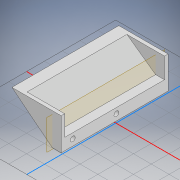
# Autodesk Inventor part: 000.001.007 - Накладка
Saved by Autodesk Inventor 2022 (Build 260153000, 153)
## iProperties
Created: 2022-11-12
Part Number: 000.001.007 - Накладка
Material: Типовые
Document SubType Name: Modeling
Designer: Petrov Ivan
Density: 1 g/cm^3
Appearance: По умолчанию
Author: Petrov Ivan
Autodesk Inventor part; units mm, degrees
ref_plane "YZ Plane" through (0, 0, 0) normal (1, 0, 0) x (0, 1, 0)
ref_plane "XZ Plane" through (0, 0, 0) normal (0, 1, 0) x (-1, 0, 0)
ref_plane "XY Plane" through (0, 0, 0) normal (0, 0, 1) x (1, 0, 0)
sketch "Эскиз1" plane through (0, 0, 0) normal (1, 0, 0) x (0, 1, 0)
  circle A0 centre (-6.0133, 48.1994) radius 2.75 projected
  circle A1 centre (-6.0133, -0.8006) radius 2.75 projected
  line L0 (-13.0133, 61.1994) -> (-13.0133, -18.8006) projected
  line L1 (38.9867, 61.1994) -> (-13.0133, 61.1994) projected
  line L2 (33.9867, -18.8006) -> (-13.0133, -18.8006) projected
  line L3 (-0.0133, 61.1994) -> (-0.0133, -18.8006)
  point P0 (0, 0)
  dimension "d0" = 13
  constraints: 2 end point, 2 point on line, 1 perpendicular
  measures "d0" distance between parallel lines of L0 L3
extrude "Выдавливание1" add sketch "Эскиз1" against normal blind 10
sketch "Эскиз2" plane through (0, -13.0133, 61.1994) normal (0, 0, 1) x (1, 0, 0)
  line L0 (-55.25, 38) -> (-55.25, 36) projected
  line L1 (-10, 13) -> (-10, 0) projected
  line L2 (-10, 0) -> (-55.25, 36)
  line L3 (0, 13) -> (-10, 13) projected
  line L4 (-10, 13) -> (-42.25, 36)
  line L5 (-55.25, 36) -> (-42.25, 36)
  point P0 (0, 13.0133)
  dimension "d3" = 13
  dimension "d4" = 13
  constraints: 6 end point, 1 horizontal
  measures "d3" distance of L1.start L1.end
  measures "d4" distance of L0.end L4.end
extrude "Выдавливание2" add sketch "Эскиз2" against normal up to surface (80 mm away)
sketch "Эскиз3" plane through (0, -13.0133, 61.1994) normal (0, 0, 1) x (1, 0, 0)
  line L0 (0, 13) -> (0, 0) projected
  line L1 (0, 13) -> (0, 36)
  line L2 (-10, 13) -> (-42.25, 36) projected
  line L3 (0, 36) -> (-42.25, 36)
  line L4 (0, 13) -> (-10, 13) projected
  point P0 (0, 13.0133)
  constraints: 4 end point, 1 perpendicular, 1 vertical
extrude "Выдавливание3" add sketch "Эскиз3" against normal blind 4
sketch "Эскиз4" plane through (-10, -6.0133, 48.1994) normal (1, 0, 0) x (0, 0, -1)
  circle A0 centre (49, 0) radius 2.75 projected
  circle A1 centre (0, 0) radius 2.75 projected
  point P0 (48.1994, 6.0133)
extrude "Выдавливание4" cut sketch "Эскиз4" against normal through all
ref_plane "РабПлоскость1" through (-10, -13.0133, 61.1994) normal (1, 0, 0) x (0, 0, 1)
sketch "Эскиз5" plane through (-10, -13.0133, 61.1994) normal (1, 0, 0) x (0, 0, 1)
  circle A0 centre (-13, -7) radius 2.75 projected
  circle A1 centre (-62, -7) radius 2.75 projected
  circle A2 centre (-13, -7) radius 2.75 projected
  circle A3 centre (-13, -7) radius 5
  circle A4 centre (-62, -7) radius 5
  point P0 (-61.1994, -13.0133)
  dimension "d12" = 10
  dimension "d13" = 10
  constraints: 2 centre point, 2 coincident
  measures "d12" diameter of A3
  measures "d13" diameter of A4
extrude "Выдавливание5" cut sketch "Эскиз5" against normal through all contours A0 | A1 | A3 | A4
move faces "Перенос2" translate (0, 0, -40) faces at (-35.8333, 10.9867, -18.8006)
sketch "Эскиз6" plane through (0, -13.0133, -58.8006) normal (0, 0, -1) x (-1, 0, 0)
  line L0 (42.25, 36) -> (10, 13) projected
  line L1 (42.25, 36) -> (0, 36) projected
  line L2 (0, 36) -> (0, 13) projected
  line L3 (10, 13) -> (0, 13) projected
  point P0 (0, 13.0133)
extrude "Выдавливание6" add sketch "Эскиз6" against normal blind 4
equation "\"d4\" = d3"
